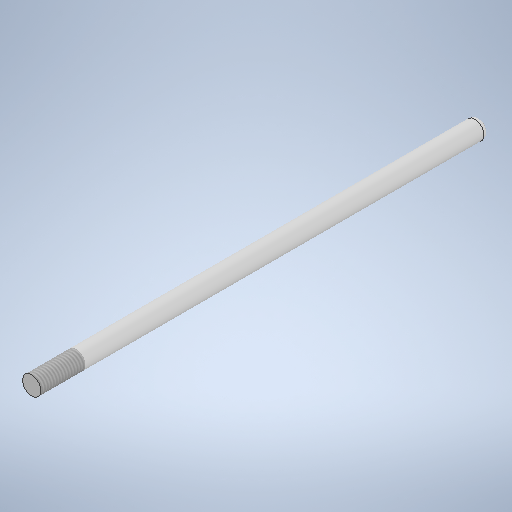
# Autodesk Inventor part: 2062
Saved by Autodesk Inventor 2025 (Build 290162010, 162A)
## iProperties
Created: 2024-05-30
Part Number: 2062
Material: Generic
Document SubType Name: Modeling
Designer: Fabri
Density: 1 g/cm^3
Appearance: Default
Author: Fabri
Autodesk Inventor part; units mm, degrees
ref_plane "YZ Plane" through (0, 0, 0) normal (1, 0, 0) x (0, 1, 0)
ref_plane "XZ Plane" through (0, 0, 0) normal (0, 1, 0) x (-1, 0, 0)
ref_plane "XY Plane" through (0, 0, 0) normal (0, 0, 1) x (1, 0, 0)
sketch "Sketch1" plane through (0, 0, 0) normal (0, 1, 0) x (-1, 0, 0)
  circle A0 centre (0, 0) radius 2.5
  dimension "d0" = 5
  constraints: 1 centre point, 1 coincident
  measures "d0" diameter of A0
extrude "Extrusion1" add sketch "Sketch1" along normal blind 121
fillet "Fillet1" radius 1.5 1 edges at (2.5, 121, 0)
thread "Thread1" size "M5x0.8" class "6g" standard "ISO Metric profile" length 12
body "Solid1"
